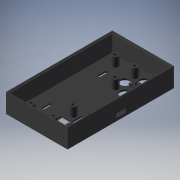
# Autodesk Inventor part: Front
Saved by Autodesk Inventor 2019 (Build 230136000, 136)
## iProperties
Created: 2020-10-05
Part Number: Front
Material: Generisch
Document SubType Name: Modeling
Designer: d_fel
Density: 1 g/cm^3
Appearance: Vorgabe
Author: d_fel
Autodesk Inventor part; units mm, degrees
ref_plane "YZ Plane" through (0, 0, 0) normal (1, 0, 0) x (0, 1, 0)
ref_plane "XZ Plane" through (0, 0, 0) normal (0, 1, 0) x (-1, 0, 0)
ref_plane "XY Plane" through (0, 0, 0) normal (0, 0, 1) x (1, 0, 0)
sketch "Skizze1" plane through (0, 0, 0) normal (0, 1, 0) x (-1, 0, 0)
  line L0 (0, 0) -> (55.8, 0)
  line L1 (55.8, 0) -> (55.8, -96.44)
  line L2 (55.8, -96.44) -> (0, -96.44)
  line L3 (0, -96.44) -> (0, 0)
  dimension "d0" = 96.44
  dimension "d1" = 55.8
  constraints: 8 end point, 2 parallel, 1 horizontal, 1 perpendicular
  measures "d0" distance of L0.end L1.end
  measures "d1" distance of L0.start L0.end
extrude "Extrusion1" add sketch "Skizze1" against normal blind 1.5
sketch "Skizze2" plane through (0, 0, 0) normal (0, 1, 0) x (1, 0, 0)
  line L0 (0, 0) -> (-55.8, 0) projected
  line L1 (-55.8, 0) -> (-55.8, 96.44) projected
  line L2 (0, 0) -> (-55.8, 0)
  line L3 (-55.8, 0) -> (-55.8, 96.44)
  line L4 (-55.8, 96.44) -> (0, 96.44)
  line L5 (0, 96.44) -> (0, 0)
  line L6 (-1.5, 1.5) -> (-54.3, 1.5)
  line L7 (-54.3, 1.5) -> (-54.3, 94.94)
  line L8 (-54.3, 94.94) -> (-1.5, 94.94)
  line L9 (-1.5, 94.94) -> (-1.5, 1.5)
  dimension "d4" = 1.5
  constraints: 16 end point, 4 parallel, 2 perpendicular, 1 horizontal, 3 other
  measures "d4" distance between parallel lines of L5 L9
extrude "Extrusion2" add sketch "Skizze2" along normal blind 15.75
sketch "Skizze4" plane through (0, 0, 0) normal (0, 1, 0) x (1, 0, 0)
  circle A0 centre (-22.82, 10.12) radius 3
  circle A1 centre (-22.82, 27.9) radius 3
  circle A2 centre (-7.58, 27.9) radius 3
  circle A3 centre (-7.58, 10.12) radius 3
  line L0 (-18.7, 6.76) -> (-18.7, 15.51)
  line L1 (-27.45, 22.51) -> (-18.7, 22.51)
  line L2 (-11.7, 15.51) -> (-11.7, 6.76)
  line L3 (-11.7, 31.26) -> (-11.7, 22.51)
  circle A4 centre (-22.82, 10.12) radius 1.3
  circle A5 centre (-22.82, 27.9) radius 1.3
  circle A6 centre (-7.58, 27.9) radius 1.3
  circle A7 centre (-7.58, 10.12) radius 1.3
  line L4 (-1.5, 1.5) -> (-54.3, 1.5) projected
  line L5 (-27.45, 22.51) -> (-27.45, 15.51)
  line L6 (-27.45, 15.51) -> (-18.7, 15.51)
  line L7 (-11.7, 22.51) -> (-2.95, 22.51)
  line L8 (-2.95, 22.51) -> (-2.95, 15.51)
  line L9 (-2.95, 15.51) -> (-11.7, 15.51)
  line L10 (-11.7, 6.76) -> (-18.7, 6.76)
  line L11 (-18.7, 22.51) -> (-18.7, 31.26)
  line L12 (-18.7, 31.26) -> (-11.7, 31.26)
  line L13 (-54.3, 1.5) -> (-54.3, 94.94) projected
  line L14 (-1.5, 94.94) -> (-1.5, 1.5) projected
  point P0 (0, 0)
  dimension "d13" = 4.12
  dimension "d15" = 4.12
  dimension "d16" = 4.12
  dimension "d17" = 6
  dimension "d18" = 6
  dimension "d19" = 6
  dimension "d20" = 6
  dimension "d21" = 2.6
  dimension "d22" = 2.6
  dimension "d23" = 2.6
  dimension "d24" = 2.6
  dimension "d25" = 17.78
  dimension "d29" = 17.78
  dimension "d30" = 15.24
  dimension "d31" = 15.24
  dimension "d32" = 4.12
  dimension "d33" = 7
  dimension "d34" = 7
  dimension "d35" = 7
  dimension "d36" = 7
  dimension "d37" = 8.75
  dimension "d38" = 8.75
  dimension "d39" = 8.75
  dimension "d40" = 8.75
  dimension "d41" = 8.75
  dimension "d42" = 8.75
  dimension "d43" = 8.75
  dimension "d44" = 8.75
  dimension "d45" = 5.39
  dimension "d46" = 8.62
  dimension "d48" = 5.39
  dimension "d147" = 6.08
  constraints: 24 end point, 8 centre point, 4 coincident, 3 perpendicular, 3 vertical, 1 horizontal, 1 parallel
  measures "d13" distance from line of L0 A0.centre
  measures "d15" distance from line of L2 A3.centre
  measures "d16" distance from line of L3 A2.centre
  measures "d17" diameter of A3
  measures "d18" diameter of A0
  measures "d19" diameter of A1
  measures "d20" diameter of A2
  measures "d21" diameter of A4
  measures "d22" diameter of A5
  measures "d23" diameter of A6
  measures "d24" diameter of A7
  measures "d25" distance of A0.centre A1.centre
  measures "d29" distance of A2.centre A3.centre
  measures "d30" distance of A3.centre A0.centre
  measures "d31" distance of A1.centre A2.centre
  measures "d32" distance from line of A1.centre L11
  measures "d33" distance of L1.start L5.end
  measures "d34" distance of L11.end L3.start
  measures "d35" distance of L2.end L0.start
  measures "d36" distance of L7.end L8.end
  measures "d37" distance of L0.start L0.end
  measures "d38" distance of L1.end L11.end
  measures "d39" distance of L3.start L3.end
  measures "d40" distance of L2.start L2.end
  measures "d41" distance of L8.end L2.start
  measures "d42" distance of L3.end L7.end
  measures "d43" distance of L1.start L1.end
  measures "d44" distance of L5.end L0.end
  measures "d45" distance from line of A4.centre L6
  measures "d46" distance from line of L4 A0.centre
  measures "d48" distance from line of L1 A1.centre
  measures "d147" distance from line of L14 A3.centre
extrude "Extrusion3" cut sketch "Skizze4" against normal blind 15 contours L0 L6 L5 L1 L11 L12 L3 L7 L8 L9 L2 L10
extrude "Extrusion4" add sketch "Skizze4" along normal blind 8.5 contours A0 | A1 | A2 | A3
sketch "Skizze5" plane through (0, 0, 0) normal (0, 1, 0) x (1, 0, 0)
  line L0 (-54.3, 1.5) -> (-54.3, 94.94) projected
  line L1 (-54.3, 94.94) -> (-1.5, 94.94) projected
  circle A0 centre (-25.36, 77.43) radius 4.5
  circle A1 centre (-7.58, 77.43) radius 4.5
  circle A2 centre (-16.47, 86.32) radius 4.5
  circle A3 centre (-16.47, 68.54) radius 4.5
  circle A4 centre (-25.36, 68.54) radius 3
  circle A5 centre (-25.36, 68.54) radius 1.35
  circle A6 centre (-25.36, 86.32) radius 3
  circle A7 centre (-25.36, 86.32) radius 1.35
  circle A8 centre (-7.58, 86.32) radius 3
  circle A9 centre (-7.58, 86.32) radius 1.35
  circle A10 centre (-7.58, 68.54) radius 3
  circle A11 centre (-7.58, 68.54) radius 1.35
  line L2 (-18.47, 74.04) -> (-18.47, 75.43)
  line L3 (-18.47, 75.43) -> (-19.86, 75.43)
  line L4 (-19.86, 75.43) -> (-19.86, 76.43)
  line L5 (-19.86, 76.43) -> (-17.47, 76.43)
  line L6 (-17.47, 76.43) -> (-17.47, 74.04)
  line L7 (-17.47, 74.04) -> (-18.47, 74.04)
  line L8 (-15.47, 74.04) -> (-15.47, 76.43)
  line L9 (-15.47, 76.43) -> (-13.08, 76.43)
  line L10 (-13.08, 76.43) -> (-13.08, 75.43)
  line L11 (-13.08, 75.43) -> (-14.47, 75.43)
  line L12 (-14.47, 75.43) -> (-14.47, 74.04)
  line L13 (-14.47, 74.04) -> (-15.47, 74.04)
  line L14 (-17.47, 78.43) -> (-17.47, 80.82)
  line L15 (-17.47, 80.82) -> (-18.47, 80.82)
  line L16 (-18.47, 80.82) -> (-18.47, 79.43)
  line L17 (-18.47, 79.43) -> (-19.86, 79.43)
  line L18 (-19.86, 79.43) -> (-19.86, 78.43)
  line L19 (-19.86, 78.43) -> (-17.47, 78.43)
  line L20 (-15.47, 78.43) -> (-13.08, 78.43)
  line L21 (-13.08, 78.43) -> (-13.08, 79.43)
  line L22 (-13.08, 79.43) -> (-14.47, 79.43)
  line L23 (-14.47, 79.43) -> (-14.47, 80.82)
  line L24 (-14.47, 80.82) -> (-15.47, 80.82)
  line L25 (-15.47, 80.82) -> (-15.47, 78.43)
  line L26 (-1.5, 94.94) -> (-1.5, 1.5) projected
  point P0 (0, 0)
  dimension "d92" = 9
  dimension "d93" = 9
  dimension "d94" = 9
  dimension "d95" = 9
  dimension "d96" = 8.62
  dimension "d98" = 8.89
  dimension "d99" = 8.89
  dimension "d100" = 8.89
  dimension "d101" = 8.89
  dimension "d102" = 6
  dimension "d103" = 2.7
  dimension "d104" = 6
  dimension "d105" = 2.7
  dimension "d106" = 6
  dimension "d107" = 2.7
  dimension "d108" = 6
  dimension "d109" = 2.7
  dimension "d110" = 8.89
  dimension "d115" = 2
  dimension "d116" = 1
  dimension "d117" = 1
  dimension "d118" = 1
  dimension "d121" = 1
  dimension "d129" = 1
  dimension "d130" = 1
  dimension "d131" = 1
  dimension "d134" = 5.5
  dimension "d135" = 5.5
  dimension "d136" = 5.5
  dimension "d137" = 5.5
  dimension "d138" = 2
  dimension "d139" = 2
  dimension "d140" = 2.39
  dimension "d141" = 2.39
  dimension "d142" = 2.39
  dimension "d143" = 1
  dimension "d144" = 2.39
  dimension "d148" = 6.08
  constraints: 48 end point, 17 perpendicular, 12 centre point, 8 point on line, 5 horizontal alignment, 4 coincident, 4 vertical alignment, 3 vertical
  measures "d92" diameter of A0
  measures "d93" diameter of A1
  measures "d94" diameter of A2
  measures "d95" diameter of A3
  measures "d96" distance from line of L1 A2.centre
  measures "d98" horizontal distance of A0.centre A2.centre
  measures "d99" horizontal distance of A0.centre A3.centre
  measures "d100" horizontal distance of A0.centre A2.centre
  measures "d101" horizontal distance of A2.centre A1.centre
  measures "d102" diameter of A4
  measures "d103" diameter of A5
  measures "d104" diameter of A6
  measures "d105" diameter of A7
  measures "d106" diameter of A8
  measures "d107" diameter of A9
  measures "d108" diameter of A10
  measures "d109" diameter of A11
  measures "d110" distance of A0.centre A4.centre
  measures "d115" distance between parallel lines of L6 L8
  measures "d116" distance between parallel lines of L12 L8
  measures "d117" distance between parallel lines of L2 L6
  measures "d118" distance between parallel lines of L5 L3
  measures "d121" distance of L9.end L10.end
  measures "d129" distance from line of L16.end L14
  measures "d130" distance of L23.end L25.start
  measures "d131" distance of L21.start L22.start
  measures "d134" distance from line of L7 A3.centre
  measures "d135" distance from line of A2.centre L15
  measures "d136" distance from line of A0.centre L18
  measures "d137" distance from line of A1.centre L21
  measures "d138" distance between parallel lines of L9 L20
  measures "d139" distance between parallel lines of L25 L14
  measures "d140" distance of L8.start L9.start
  measures "d141" distance of L4.end L5.end
  measures "d142" distance of L19.start L19.end
  measures "d143" distance from line of L6 A3.centre
  measures "d144" distance of L9.start L9.end
  measures "d148" distance from line of L26 A8.centre
extrude "Extrusion5" cut sketch "Skizze5" against normal blind 15 contours A0 | A1 | A2 | A3
extrude "Extrusion6" add sketch "Skizze5" along normal blind 8.5 contours A4 | A6 | A8 | A10
extrude "Extrusion7" add sketch "Skizze5" along normal blind 3 contours L2 L3 L4 L5 L6 L7 | L8 L9 L10 L11 L12 L13 | L19 L18 L17 L16 L15 L14 | L25 L24 L23 L22 L21 L20
sketch "Skizze6" plane through (0, 0, 0) normal (0, 1, 0) x (1, 0, 0)
  line L0 (-43.12, 19.57) -> (-43.12, 26.07)
  line L1 (-40.62, 26.07) -> (-40.62, 19.57)
  arc A0 (-43.12, 19.57) -> (-40.62, 19.57) centre (-41.87, 19.57) ccw
  arc A1 (-40.62, 26.07) -> (-43.12, 26.07) centre (-41.87, 26.07) ccw
  circle A2 centre (-22.82, 27.9) radius 1.3 projected
  line L2 (-43.12, 70.37) -> (-43.12, 76.87)
  line L3 (-40.62, 76.87) -> (-40.62, 70.37)
  arc A3 (-43.12, 70.37) -> (-40.62, 70.37) centre (-41.87, 70.37) ccw
  arc A4 (-40.62, 76.87) -> (-43.12, 76.87) centre (-41.87, 76.87) ccw
  circle A5 centre (-25.36, 86.32) radius 1.35 projected
  circle A6 centre (-25.36, 68.54) radius 1.35 projected
  point P0 (0, 0)
  dimension "d149" = 6.5
  dimension "d150" = 2.5
  dimension "d151" = 19.05
  dimension "d152" = 1.83
  dimension "d153" = 6.5
  dimension "d154" = 2.5
  dimension "d156" = 16.51
  dimension "d157" = 1.83
  constraints: 8 end point, 8 point on circle, 8 tangent, 4 centre point, 2 vertical
  measures "d149" distance of L1.start L1.end
  measures "d150" distance between parallel lines of L0 L1
  measures "d151" horizontal distance of A1.centre A2.centre
  measures "d152" vertical distance of A1.centre A2.centre
  measures "d153" distance of L3.start L3.end
  measures "d154" distance between parallel lines of L2 L3
  measures "d156" horizontal distance of A6.centre A3.centre
  measures "d157" vertical distance of A3.centre A6.centre
extrude "Extrusion8" cut sketch "Skizze6" against normal blind 3 contours L0 A1 L1 A0 | L2 A4 L3 A3
sketch "Skizze7" plane through (0, 0, 0) normal (0, 1, 0) x (1, 0, 0)
  circle A0 centre (-43.14, 86.32) radius 3
  circle A1 centre (-43.14, 10.12) radius 3
  circle A2 centre (-43.14, 86.32) radius 1.35
  circle A3 centre (-43.14, 10.12) radius 1.35
  line L0 (-1.5, 1.5) -> (-54.3, 1.5) projected
  line L1 (-1.5, 94.94) -> (-1.5, 1.5) projected
  circle A4 centre (-25.36, 86.32) radius 1.35 projected
  circle A5 centre (-22.82, 10.12) radius 1.3 projected
  point P0 (0, 0)
  dimension "d160" = 6
  dimension "d161" = 6
  dimension "d162" = 2.7
  dimension "d163" = 2.7
  dimension "d167" = 0
  dimension "d168" = 0
  dimension "d169" = 17.78
  dimension "d170" = 20.32
  constraints: 4 centre point, 2 coincident
  measures "d160" diameter of A0
  measures "d161" diameter of A1
  measures "d162" diameter of A3
  measures "d163" diameter of A2
  measures "d167" vertical distance of A4.centre A0.centre
  measures "d168" vertical distance of A5.centre A1.centre
  measures "d169" distance of A4.centre A0.centre
  measures "d170" distance of A1.centre A5.centre
extrude "Extrusion9" add sketch "Skizze7" along normal blind 8.5 contours A0 | A1
sketch "Skizze9" plane through (0, -1.5, 0) normal (1, 0, 0) x (0, 0, -1)
  line L0 (44.47, 6) -> (52.97, 6)
  line L1 (52.97, 6) -> (52.97, 2.5)
  line L2 (52.97, 2.5) -> (44.47, 2.5)
  line L3 (44.47, 2.5) -> (44.47, 6)
  line L4 (1.5, 1.5) -> (94.94, 1.5) projected
  line L5 (0, 0) -> (0, 17.25) projected
  point P0 (0, 1.5)
  dimension "d173" = 4.5
  dimension "d174" = 1
  dimension "d175" = 8.5
  dimension "d177" = 44.47
  constraints: 8 end point, 2 parallel, 1 horizontal, 1 perpendicular
  measures "d173" distance between parallel lines of L4 L0
  measures "d174" distance between parallel lines of L2 L4
  measures "d175" distance of L1.end L2.end
  measures "d177" distance between parallel lines of L3 L5
extrude "Extrusion10" cut sketch "Skizze9" against normal blind 8.5
sketch "Skizze14" plane through (0, 15.75, 0) normal (0, 1, 0) x (1, 0, 0)
  line L0 (-1.5, 1.5) -> (-54.3, 1.5) projected
  line L1 (-1.5, 1.5) -> (-1.5, 94.94) projected
  line L2 (-54.3, 1.5) -> (-1.5, 1.5)
  line L3 (-1.5, 1.5) -> (-1.5, 94.94)
  line L4 (-1.5, 94.94) -> (-54.3, 94.94)
  line L5 (-54.3, 94.94) -> (-54.3, 1.5)
  line L6 (-55.05, 95.69) -> (-0.75, 95.69)
  line L7 (-0.75, 95.69) -> (-0.75, 0.75)
  line L8 (-0.75, 0.75) -> (-55.05, 0.75)
  line L9 (-55.05, 0.75) -> (-55.05, 95.69)
  point P0 (0, 0)
  dimension "d180" = 0.75
  constraints: 16 end point, 4 parallel, 2 perpendicular, 1 horizontal, 3 other
  measures "d180" distance between parallel lines of L4 L6
extrude "Extrusion11" cut sketch "Skizze14" against normal blind 0.75
